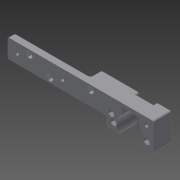
# Autodesk Inventor part: Base
Saved by Autodesk Inventor 2015 (Build 190159000, 159)
## iProperties
Created: 2017-07-05
Part Number: Base
Material: Generic
Document SubType Name: Modeling
Designer: Bruno
Density: 1 g/cm^3
Appearance: Default
Author: Bruno
Autodesk Inventor part; units mm, degrees
ref_plane "YZ Plane" through (0, 0, 0) normal (1, 0, 0) x (0, 1, 0)
ref_plane "XZ Plane" through (0, 0, 0) normal (0, 1, 0) x (-1, 0, 0)
ref_plane "XY Plane" through (0, 0, 0) normal (0, 0, 1) x (1, 0, 0)
sketch "Sketch1" plane through (0, 0, 0) normal (0, 1, 0) x (-1, 0, 0)
  circle A0 centre (17.5, 0) radius 2
  circle A1 centre (-17.5, 0) radius 2
  line L0 (-25, 22) -> (-25, -8)
  line L1 (25, -8) -> (25, 8)
  line L2 (-25, 22) -> (25, 22)
  line L3 (25, 22) -> (25, 8)
  line L4 (9, 18) -> (9, 10.7238)
  line L5 (-9, 18) -> (-9, 10.7238)
  arc A2 (-9, 10.7238) -> (-11.4891, -8) centre (0, 0) ccw
  arc A3 (11.4891, -8) -> (9, 10.7238) centre (0, 0) ccw
  line L6 (11.4891, -8) -> (25, -8)
  line L7 (9, 18) -> (-9, 18)
  line L8 (-11.4891, -8) -> (-25, -8)
  dimension "d3" = 4
  dimension "d4" = 4
  dimension "d7" = 50
  constraints: 18 end point, 4 centre point, 4 point on circle, 2 horizontal, 2 parallel, 2 vertical, 1 coincident
  measures "d3" diameter of A0
  measures "d4" diameter of A1
  measures "d7" distance of L1.start L0.end
extrude "Extrusion1" add sketch "Sketch1" along normal blind 20
sketch "Sketch2" plane through (0, 0, 0) normal (0, 1, 0) x (-1, 0, 0)
  circle A0 centre (-17.5, 0) radius 2 projected
  circle A1 centre (17.5, 0) radius 2 projected
  line L0 (9, 18) -> (9, 10.7238) projected
  arc A2 (11.4891, -8) -> (9, 10.7238) centre (0, 0) ccw projected
  line L1 (11.4891, -8) -> (25, -8) projected
  line L2 (25, -8) -> (25, 22) projected
  line L3 (25, 22) -> (-25, 22) projected
  line L4 (-25, 22) -> (-25, -8) projected
  line L5 (-25, -8) -> (-11.4891, -8) projected
  arc A3 (-9, 10.7238) -> (-11.4891, -8) centre (0, 0) ccw projected
  line L6 (-9, 10.7238) -> (-9, 18) projected
  line L7 (-9, 18) -> (9, 18) projected
  line L8 (25, 22) -> (50, 22)
  line L9 (50, 22) -> (50, 2)
  line L10 (50, 2) -> (25, 2)
  line L11 (25, 2) -> (25, 22)
  dimension "d12" = 25
  dimension "d13" = 20
  constraints: 8 end point, 2 parallel, 1 horizontal, 1 perpendicular
  measures "d12" distance of L9.end L10.end
  measures "d13" distance of L8.end L9.end
extrude "Extrusion2" add sketch "Sketch2" along normal blind 20 contours L2 L8 L9 L10
sketch "Sketch4" plane through (0, 0, 0) normal (0, 1, 0) x (-1, 0, 0)
  line L0 (50, 2) -> (130, 2)
  line L1 (130, 2) -> (130, 22)
  line L2 (130, 22) -> (50, 22)
  line L3 (50, 22) -> (50, 2)
  point P0 (0, 0)
  dimension "d18" = 80
  constraints: 8 end point, 2 parallel, 1 horizontal, 1 perpendicular
  measures "d18" distance of L2.end L1.end
extrude "Extrusion3" add sketch "Sketch4" along normal blind 8
sketch "Sketch5" plane through (0, 20, 0) normal (0, 1, 0) x (1, 0, 0)
  line L0 (0, 0) -> (0, 8)
  line L1 (0, 8) -> (-50, 8)
  line L2 (-50, 8) -> (-50, -2)
  line L3 (-50, -2) -> (0, -2)
  line L4 (0, -2) -> (0, 8)
  line L5 (-50, -2) -> (0, -2)
  line L6 (0, -2) -> (0, -4)
  line L7 (0, -4) -> (-50, -4)
  line L8 (-50, -4) -> (-50, -2)
  line L9 (-50, -22) -> (25, -22) projected
  line L10 (-50, -4) -> (-45, -4)
  line L11 (-45, -4) -> (-45, -22)
  line L12 (-45, -22) -> (-50, -22)
  line L13 (-50, -22) -> (-50, -4)
  circle A0 centre (-17.5, 0) radius 2 projected
  circle A1 centre (-17.5, 0) radius 3.5
  line L14 (-45, -4) -> (-17, -4)
  line L15 (-17, -4) -> (-17, -20)
  line L16 (-17, -20) -> (-45, -20)
  line L17 (-45, -20) -> (-45, -4)
  arc A2 (-11.4891, 8) -> (-9, -10.7238) centre (0, 0) ccw projected
  line L18 (-17, -4) -> (-20, -4)
  line L19 (-17, -7) -> (-17, -4)
  line L20 (-45, -20) -> (-42, -20)
  line L21 (-45, -17) -> (-45, -20)
  circle A3 centre (-42, -17) radius 1.7
  circle A4 centre (-20, -7) radius 1.7
  dimension "d21" = 8
  dimension "d22" = 10
  dimension "d23" = 2
  dimension "d24" = 5
  dimension "d25" = 7
  dimension "d26" = 28
  dimension "d27" = 16
  dimension "d32" = 3.4
  dimension "d33" = 3.4
  constraints: 42 end point, 8 parallel, 6 horizontal, 4 perpendicular, 3 centre point, 1 coincident, 1 point on line, 1 vertical
  measures "d21" distance of L0.start L0.end
  measures "d22" distance of L2.end L1.end
  measures "d23" distance of L5.end L6.end
  measures "d24" distance of L11.end L12.end
  measures "d25" diameter of A1
  measures "d26" distance of L15.end L16.end
  measures "d27" distance of L14.end L15.end
  measures "d32" diameter of A3
  measures "d33" diameter of A4
extrude "Extrusion4" cut sketch "Sketch5" against normal blind 1 contours L15 L16 L11 L7
sketch "Sketch6" plane through (-42, 20, 17) normal (0, 1, 0) x (1, 0, 0)
  circle A0 centre (0, 0) radius 1.7 projected
  circle A1 centre (22, 10) radius 1.7 projected
  point P0 (42, 17)
extrude "Extrusion5" cut sketch "Sketch6" against normal blind 20
sketch "Sketch7" plane through (0, 8, 0) normal (0, 1, 0) x (1, 0, 0)
  line L0 (-50, -2) -> (-130, -2) projected
  line L1 (-130, -2) -> (-130, -22) projected
  line L2 (-130, -22) -> (-50, -22) projected
  line L3 (-50, -2) -> (-50, -22) projected
  circle A0 centre (-20, -7) radius 1.7 projected
  circle A1 centre (-42, -17) radius 1.7 projected
  line L4 (-45, -20) -> (-45, -4) projected
  line L5 (-17, -20) -> (-45, -20) projected
  line L6 (-17, -4) -> (-17, -20) projected
  line L7 (-45, -4) -> (-17, -4) projected
  line L8 (-45, -4) -> (-130, -4)
  line L9 (-130, -2) -> (-130, -22) projected
  line L10 (-130, -22) -> (25, -22) projected
  line L11 (-130, -2) -> (-115, -2)
  line L12 (-115, -2) -> (-115, -22)
  line L13 (-115, -22) -> (-130, -22)
  line L14 (-130, -22) -> (-130, -2)
  line L15 (-17, -4) -> (-17, -20)
  line L16 (-17, -20) -> (-45, -20)
  circle A2 centre (-42, -17) radius 1.7
  circle A3 centre (-20, -7) radius 1.7
  circle A4 centre (-85, -7) radius 1.7
  line L17 (-110, -20) -> (-110, -4)
  line L18 (-82, -20) -> (-110, -20)
  line L19 (-82, -4) -> (-82, -20)
  line L20 (-110, -4) -> (-82, -4)
  circle A5 centre (-107, -17) radius 1.7
  line L21 (-130, -4) -> (-110, -4)
  point P0 (0, 0)
  dimension "d38" = 15
  dimension "d39" = 28
  dimension "d40" = 16
  dimension "d41" = 3.4
  dimension "d42" = 3.4
  dimension "d43" = 3.4
  dimension "d44" = 20
  constraints: 24 end point, 4 centre point, 3 point on line, 2 parallel, 2 perpendicular, 1 horizontal
  measures "d38" distance of L12.end L13.end
  measures "d39" distance of L16.start L16.end
  measures "d40" distance of L15.start L16.start
  measures "d41" diameter of A2
  measures "d42" diameter of A3
  measures "d43" diameter of A5
  measures "d44" distance of L8.end L21.end
extrude "Extrusion6" cut sketch "Sketch7" against normal blind 1 contours L19 L18 L17 L8
sketch "Sketch8" plane through (-107, 8, 17) normal (0, 1, 0) x (1, 0, 0)
  circle A0 centre (0, 0) radius 1.7 projected
  circle A1 centre (22, 10) radius 1.7 projected
  point P0 (107, 17)
extrude "Extrusion7" cut sketch "Sketch8" against normal blind 8
sketch "Sketch9" plane through (0, 0, 0) normal (0, -1, 0) x (1, 0, 0)
  circle A0 centre (-107, 17) radius 1.7 projected
  circle A1 centre (-85, 7) radius 1.7 projected
  circle A2 centre (-42, 17) radius 1.7 projected
  circle A3 centre (-20, 7) radius 1.7 projected
  circle A4 centre (17.5, 0) radius 2 projected
  circle A5 centre (-17.5, 0) radius 2 projected
  line L0 (-9, 18) -> (-9, 10.7238) projected
  line L1 (9, 18) -> (-9, 18) projected
  line L2 (9, 10.7238) -> (9, 18) projected
  arc A6 (11.4891, -8) -> (9, 10.7238) centre (0, 0) ccw projected
  line L3 (25, -8) -> (11.4891, -8) projected
  line L4 (25, 22) -> (25, -8) projected
  line L5 (-130, 22) -> (25, 22) projected
  line L6 (-130, 2) -> (-130, 22) projected
  line L7 (-25, 2) -> (-130, 2) projected
  line L8 (-25, -8) -> (-25, 2) projected
  line L9 (-11.4891, -8) -> (-25, -8) projected
  arc A7 (-9, 10.7238) -> (-11.4891, -8) centre (0, 0) ccw projected
  circle A8 centre (-107, 17) radius 3
  circle A9 centre (-85, 7) radius 1.7 projected
  circle A10 centre (-85, 7) radius 3
  circle A11 centre (-42, 17) radius 3
  circle A12 centre (-17.5, 0) radius 3
  circle A13 centre (17.5, 0) radius 3
  line L10 (-82, 20) -> (-110, 20) projected
  line L11 (-105.2679, 20) -> (-103.5359, 17)
  line L12 (-103.5359, 17) -> (-105.2679, 14)
  line L13 (-105.2679, 14) -> (-108.7321, 14)
  line L14 (-108.7321, 14) -> (-110.4641, 17)
  line L15 (-110.4641, 17) -> (-108.7321, 20)
  line L16 (-108.7321, 20) -> (-105.2679, 20)
  line L17 (-83.2679, 10) -> (-81.5359, 7)
  line L18 (-81.5359, 7) -> (-83.2679, 4)
  line L19 (-83.2679, 4) -> (-86.7321, 4)
  line L20 (-86.7321, 4) -> (-88.4641, 7)
  line L21 (-88.4641, 7) -> (-86.7321, 10)
  line L22 (-86.7321, 10) -> (-83.2679, 10)
  line L23 (-40.2679, 20) -> (-38.5359, 17)
  line L24 (-38.5359, 17) -> (-40.2679, 14)
  line L25 (-40.2679, 14) -> (-43.7321, 14)
  line L26 (-43.7321, 14) -> (-45.4641, 17)
  line L27 (-45.4641, 17) -> (-43.7321, 20)
  line L28 (-43.7321, 20) -> (-40.2679, 20)
  line L29 (-14.5, -1.7321) -> (-17.5, -3.4641)
  line L30 (-17.5, -3.4641) -> (-20.5, -1.7321)
  line L31 (-20.5, -1.7321) -> (-20.5, 1.7321)
  line L32 (-20.5, 1.7321) -> (-17.5, 3.4641)
  line L33 (-17.5, 3.4641) -> (-14.5, 1.7321)
  line L34 (-14.5, 1.7321) -> (-14.5, -1.7321)
  circle A14 centre (-20, 7) radius 1.7 projected
  circle A15 centre (-20, 7) radius 3
  line L35 (-17, 4) -> (-17, 20) projected
  line L36 (-17, 5.2679) -> (-20, 3.5359)
  line L37 (-20, 3.5359) -> (-23, 5.2679)
  line L38 (-23, 5.2679) -> (-23, 8.7321)
  line L39 (-23, 8.7321) -> (-20, 10.4641)
  line L40 (-20, 10.4641) -> (-17, 8.7321)
  line L41 (-17, 8.7321) -> (-17, 5.2679)
  line L42 (20.5, -1.7321) -> (17.5, -3.4641)
  line L43 (17.5, -3.4641) -> (14.5, -1.7321)
  line L44 (14.5, -1.7321) -> (14.5, 1.7321)
  line L45 (14.5, 1.7321) -> (17.5, 3.4641)
  line L46 (17.5, 3.4641) -> (20.5, 1.7321)
  line L47 (20.5, 1.7321) -> (20.5, -1.7321)
  point P0 (-107, 20)
  point P1 (-85, 10)
  point P2 (-42, 20)
  point P3 (-14.5, 0)
  point P4 (-17, 7)
  point P5 (20.5, 0)
  dimension "d49" = 6
  dimension "d50" = 6
  dimension "d51" = 6
  dimension "d53" = 6
  dimension "d54" = 6
  dimension "d55" = 6
  constraints: 72 end point, 12 coincident, 6 midpoint, 3 horizontal alignment, 3 point on line, 3 vertical alignment, 90 other
extrude "Extrusion8" cut sketch "Sketch9" against normal blind 4 contours A8 | A8 L11 L12 | A8 L10 L11 | L12 L13 A8 | A8 L15 L10 | L13 L14 A8 | A8 L14 L15 | A10 | A10 L17 L18 | A10 L22 L17 | L18 L19 A10 | A10 L21 L22 | L19 L20 A10 | A10 L20 L21 | A11 | A11 L23 L24 | A11 L28 L23 | L24 L25 A11 | A11 L27 L28 | L25 L26 A11 | A11 L26 L27 | A12 | L34 L29 A12 | A12 L33 L34 | A12 L32 L33 | L29 L30 A12 | A12 L31 L32 | L30 L31 A12 | A13 | L47 L42 A13 | A13 L46 L47 | A13 L45 L46 | L42 L43 A13 | A13 L44 L45 | L43 L44 A13 | A15 | L35 L36 A15 | A15 L40 L35 | A15 L39 L40 | L36 L37 A15 | A15 L38 L39 | L37 L38 A15
sketch "Sketch10" plane through (0, 20, 0) normal (0, 1, 0) x (1, 0, 0)
  line L0 (9, -18) -> (-9, -18) projected
  line L1 (-50, -22) -> (25, -22) projected
  line L2 (-9, -22) -> (-9, -18)
  line L3 (9, -10.7238) -> (9, -18) projected
  arc A0 (9, -10.7238) -> (11.4891, 8) centre (0, 0) ccw projected
  line L4 (25, 8) -> (11.4891, 8) projected
  line L5 (25, -22) -> (25, 8) projected
  line L6 (9, -18) -> (9, -22)
  constraints: 4 end point, 3 point on line, 1 perpendicular
extrude "Extrusion9" cut sketch "Sketch10" against normal blind 4 contours L6 L1 L2 L0
fillet "Fillet1" radius 2 24 edges at (-25, 10, -8) (25, 10, -8) (25, 10, 22) (-50, 14, 2) (-130, 4, 2) (-50, 14, 22) (-130, 4, 22) (9, 18, 22) (-9, 18, 22) (0, 16, 22) (-29.5, 20, 22) (-37.5, 20, 2) (-25, 20, -3) (-18.2446, 20, -8) (17, 20, 22) (25, 20, 7) (18.2446, 20, -8) (-50, 20, 12) (-50, 8, 12) (-90, 8, 22) (-90, 8, 2) (-130, 8, 12) (-9, 20, 16.3619) (9, 20, 16.3619)
sketch "Sketch11" plane through (0, 8, 0) normal (0, 1, 0) x (1, 0, 0)
  line L0 (-82, -4) -> (-82, -20) projected
  line L1 (-110, -20) -> (-110, -4) projected
  line L2 (-130, -2) -> (-130, -22) projected
  line L3 (-130, -12) -> (-110, -12)
  circle A0 centre (-120, -12) radius 2
  line L4 (-82, -12) -> (-72, -12)
  circle A1 centre (-72, -12) radius 2
  line L5 (-82, -4) -> (-52, -4) projected
  line L6 (-52, -20) -> (-82, -20) projected
  line L7 (-52, -4) -> (-52, -20) projected
  line L8 (-128, -4) -> (-110, -4) projected
  line L9 (-128, -20) -> (-128, -4) projected
  line L10 (-110, -20) -> (-128, -20) projected
  point P0 (0, 0)
  dimension "d61" = 4
  dimension "d62" = 10
  dimension "d63" = 4
  constraints: 4 end point, 4 midpoint, 2 centre point, 1 coincident, 1 point on line
  measures "d61" diameter of A0
  measures "d62" distance of L4.start L4.end
  measures "d63" diameter of A1
extrude "Extrusion10" cut sketch "Sketch11" against normal blind 8 contours A0 L3 | L3 A0 | A1
sketch "Sketch13" plane through (0, 20, 0) normal (0, 1, 0) x (1, 0, 0)
  line L0 (9, -10.7238) -> (9, -18) projected
  line L1 (9, -14.3619) -> (25, -14.3619)
  line L2 (25, -22) -> (25, 8) projected
  line L3 (9, -14.3619) -> (25, -14.3619) construction
  circle A0 centre (17, -14.3619) radius 2
  point P0 (0, 0)
  dimension "d67" = 0
  dimension "d68" = 4
  constraints: 4 end point, 2 midpoint, 1 centre point, 1 collinear, 1 horizontal, 1 point on line
  measures "d67" distance between parallel lines of L1 L3
  measures "d68" diameter of A0
extrude "Extrusion11" cut sketch "Sketch13" against normal blind 20
chamfer "Chamfer1" distance 1 angle 45 3 edges at (15, 20, 14.3619) (-74, 8, 12) (-122, 8, 12)
body "Solid1"
